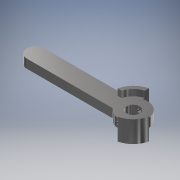
# Autodesk Inventor part: Handle
Saved by Autodesk Inventor 2018 (Build 220112000, 112)
## iProperties
Shininess: 64.0
Length Units: 11269
Angle Units: 11279
Time Units: 11290
Mass Units: 11283
Length Display Precision: 3
Angle Display Precision: 2
Compacted: True
Part Number: Handle
Document SubType Name: Modeling
Created: 2003-04-19
Designer: James M. Leake
Material: Steel, Mild
Density: 7.85 g/cm^3
Appearance: Semi-Polished
Density: 0.0
Volumn: 0.0
Area: 0.0
PropertySet Name: Model Information
Control State: 0
Master: False
Checked Out: False
Author: James M. Leake
Autodesk Inventor part; units mm, degrees
ref_plane "YZ Plane" through (0, 0, 0) normal (1, 0, 0) x (0, 1, 0)
ref_plane "XZ Plane" through (0, 0, 0) normal (0, 1, 0) x (-1, 0, 0)
ref_plane "XY Plane" through (0, 0, 0) normal (0, 0, 1) x (1, 0, 0)
sketch "Sketch1" plane through (0, 0, 0) normal (0, 0, 1) x (1, 0, 0)
  line L0 (-122.1855, 0) -> (62.4119, 0) projected
  line L1 (0, -27.4264) -> (0, 36.5685) projected
  circle A0 centre (0, 0) radius 6.5
  line L2 (-4.5, 20.5122) -> (-4.5, 14.3091)
  line L3 (-20.5122, 4.5) -> (-14.3091, 4.5)
  line L4 (4.5, -14.3091) -> (4.5, -20.5122)
  line L5 (20.5122, -4.5) -> (14.3091, -4.5)
  arc A1 (-4.5, 20.5122) -> (-20.5122, 4.5) centre (0, 0) ccw
  arc A2 (4.5, -20.5122) -> (20.5122, -4.5) centre (0, 0) ccw
  arc A3 (-4.5, 16.3936) -> (-16.3936, 4.5) centre (0, 0) ccw
  arc A4 (4.5, -16.3936) -> (16.3936, -4.5) centre (0, 0) ccw
  arc A5 (-14.3091, 4.5) -> (4.5, -14.3091) centre (0, 0) ccw
  arc A6 (14.3091, -4.5) -> (-4.5, 14.3091) centre (0, 0) ccw
  line L6 (-18.9737, 9) -> (-100, 9)
  arc A7 (-100, 9) -> (-100, -9) centre (-100, 0) ccw
  line L7 (-100, -9) -> (-12, -9)
  dimension "d0" = 13
  dimension "d1" = 30
  dimension "d2" = 34
  dimension "d3" = 42
  dimension "d4" = 4.5
  dimension "d5" = 4.5
  dimension "d6" = 100
  dimension "d7" = 9
  constraints: 16 point on circle, 12 end point, 8 centre point, 5 parallel, 4 point on line, 3 concentric, 3 perpendicular, 2 tangent, 1 coincident, 1 other
  measures "d0" diameter of A0
  measures "d1" diameter of A6
  measures "d2" diameter of A4
  measures "d3" diameter of A2
  measures "d4" distance between parallel lines of L1 L2
  measures "d5" distance between parallel lines of L5 L0
  measures "d6" distance from line of A7.centre L1
  measures "d7" radius of A7
extrude "Extrusion1" add sketch "Sketch1" along normal mid plane 9 contours A7 L6 A1 L3 A5 L0 | L0 A5 L7 A7 | A5 L3 A3 L2 A6 L1 A0 L0 | L0 A0 L1 A5 | L1 A6 L0 A0 | A0 L0 A6 L5 A4 L4 A5 L1
extrude "Extrusion2" add sketch "Sketch1" along normal mid plane 22 contours A1 L2 A3 L3 | A4 L5 A2 L4
sketch "Sketch2" plane through (0, 0, 0) normal (0, 1, 0) x (-1, 0, 0)
  line L0 (2.4, 0) -> (-3.2, 0) projected
  line L1 (0, -2.4) -> (0, 3.2) projected
  circle A0 centre (0, 0) radius 2
  dimension "d12" = 4
  constraints: 1 centre point, 1 coincident
  measures "d12" diameter of A0
extrude "Extrusion3" cut sketch "Sketch2" along normal through all both and the other way through all
body "Solid1"
